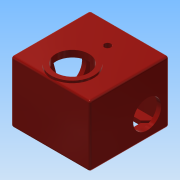
# Autodesk Inventor part: кожух  блока
Saved by Autodesk Inventor 2017 (Build 210142000, 142)
## iProperties
Part Number: кожух  блока
Material: Типовые
Document SubType Name: Modeling
Designer: Max
Mass: 1.18603 g
Surface Area: 24.9841 cm^2
Volume: 1.18603 cm^3
Density: 1 g/cm^3
Appearance: Оранжево-красный
Author: Max
Autodesk Inventor part; units mm, degrees
ref_plane "YZ Plane" through (0, 0, 0) normal (1, 0, 0) x (0, 1, 0)
ref_plane "XZ Plane" through (0, 0, 0) normal (0, 1, 0) x (-1, 0, 0)
ref_plane "XY Plane" through (0, 0, 0) normal (0, 0, 1) x (1, 0, 0)
sketch "Эскиз1" plane through (0, 0, 0) normal (0, 0, 1) x (1, 0, 0)
  line L0 (-8, -8) -> (8, -8)
  line L1 (8, -8) -> (8, 8)
  line L2 (8, 8) -> (-8, 8)
  line L3 (-8, 8) -> (-8, -8)
  circle A0 centre (0, -4) radius 2.3157
  circle A1 centre (0, 4) radius 0.75
  line L4 (-9, -9) -> (9, -9)
  line L5 (9, -9) -> (9, 9)
  line L6 (9, 9) -> (-9, 9)
  line L7 (-9, 9) -> (-9, -9)
  point P0 (0, 0)
  dimension "d0" = 16
  dimension "d1" = 16
  dimension "d2" = 8
  dimension "d3" = 8
  dimension "d4" = 1.5
  dimension "d5" = 4
  dimension "d6" = 4
  dimension "d7" = 1
  constraints: 16 end point, 4 parallel, 2 centre point, 2 perpendicular, 1 horizontal, 3 other
  measures "d0" distance between parallel lines of L1 L3
  measures "d1" distance between parallel lines of L2 L0
  measures "d2" distance from line of L0 point (0, 0)
  measures "d3" distance from line of L3 point (0, 0)
  measures "d4" diameter of A1
  measures "d5" distance from line of L0 A0.centre
  measures "d6" distance from line of L2 A1.centre
  measures "d7" distance between parallel lines of L3 L7
extrude "Выдавливание1" add sketch "Эскиз1" along normal blind 1 contours L3 L2 L1 L0 | L7 L6 L5 L4
extrude "Выдавливание2" add sketch "Эскиз1" against normal blind 13 contours L7 L6 L5 L4
sketch "Эскиз2" plane through (0, 0, -13) normal (0, 0, -1) x (-1, 0, 0)
  line L0 (-8, -8) -> (-8, 8)
  line L1 (-8, 8) -> (8, 8)
  line L2 (8, 8) -> (8, -8)
  line L3 (8, -8) -> (-8, -8)
  line L4 (-9, -9) -> (9, -9)
  line L5 (9, -9) -> (9, 9)
  line L6 (9, 9) -> (-9, 9)
  line L7 (-9, 9) -> (-9, -9)
  line L8 (-6, 5.5) -> (-6, -5.5)
  line L9 (6, -5.5) -> (6, 5.5)
  line L10 (5.5, 6) -> (-5.5, 6)
  spline S0 degree 3 number of poles 196 construction
  circle A0 centre (0, -4) radius 2.3157
  arc A1 (-1.5842, -6) -> (1.5842, -6) centre (0, -4) ccw
  line L11 (-5.5, -6) -> (-1.5842, -6)
  line L12 (-1.1537, -6) -> (-1.1341, -6)
  line L13 (1.5842, -6) -> (5.5, -6)
  line L14 (1.1397, -6) -> (1.1535, -6)
  line L15 (-8, -8) -> (8, -8) construction
  line L16 (-8, -8) -> (8, 8) construction
  line L17 (8, 8) -> (-8, 8) construction
  line L18 (-8, 8) -> (8, -8) construction
  line L19 (7.0273, 7.0273) -> (-7.0273, 7.0273) construction
  line L20 (-7.0273, 7.0273) -> (-7.0273, -7.0273) construction
  line L21 (-7.0273, -7.0273) -> (7.0273, -7.0273) construction
  line L22 (7.0273, -7.0273) -> (7.0273, 7.0273) construction
  line L23 (7.0273, 7.0273) -> (-7.0273, -7.0273) construction
  line L24 (-7.0273, 7.0273) -> (7.0273, -7.0273) construction
  arc A2 (-7.0273, -6.5273) -> (-6.5273, -7.0273) centre (-7.0273, -7.0273) ccw
  arc A3 (-6.5273, 7.0273) -> (-7.0273, 6.5273) centre (-7.0273, 7.0273) ccw
  arc A4 (7.0273, 6.5273) -> (6.5273, 7.0273) centre (7.0273, 7.0273) ccw
  arc A5 (6.5273, -7.0273) -> (7.0273, -6.5273) centre (7.0273, -7.0273) ccw
  line L25 (-6, -5.5) -> (-7.0273, -6.5273)
  line L26 (-6.5273, -7.0273) -> (-5.5, -6)
  line L27 (-6, 5.5) -> (-7.0273, 6.5273)
  line L28 (-6.5273, 7.0273) -> (-5.5, 6)
  line L29 (6.5273, -7.0273) -> (5.5, -6)
  line L30 (0, -0.5) -> (-0.5, 0)
  line L31 (0, 0.5) -> (0.5, 0)
  line L32 (6, -5.5) -> (7.0273, -6.5273)
  line L33 (0, -0.5) -> (0.5, 0)
  line L34 (6, 5.5) -> (7.0273, 6.5273)
  line L35 (6.5273, 7.0273) -> (5.5, 6)
  line L36 (0, 0.5) -> (-0.5, 0)
  point P0 (0, 0)
  dimension "d12" = 2
  dimension "d16" = 1
  dimension "d17" = 1
  dimension "d18" = 1
  dimension "d19" = 1
  constraints: 54 end point, 10 point on circle, 9 point on line, 5 centre point, 5 coincident, 2 midpoint, 2 parallel, 2 perpendicular, 1 horizontal, 4 other
  measures "d12" distance between parallel lines of L0 L8
  measures "d16" diameter of A2
  measures "d17" diameter of A3
  measures "d18" diameter of A4
  measures "d19" diameter of A5
extrude "Выдавливание3" add sketch "Эскиз2" against normal blind 1 contours L0 L1 L2 L3
fillet "Сопряжение1" radius 0.5 12 edges at (9, -9, -6) (-9, -9, -6) (-9, 9, -6) (9, 9, -6) (-9, 0, 1) (0, -9, 1) (0, 9, 1) (9, 0, 1) (0, 9, -13) (9, 0, -13) (0, -9, -13) (-9, 0, -13)
sketch "Эскиз3" plane through (0, 0, 1) normal (0, 0, 1) x (1, 0, 0)
  circle A0 centre (0, -4) radius 2.3157 projected
  circle A1 centre (0, -4) radius 2.3157
  circle A2 centre (0, -4) radius 3.75
  circle A3 centre (0, -4) radius 4.8299
  point P0 (0, 0)
  dimension "d22" = 7.5
  constraints: 3 centre point, 2 coincident
  measures "d22" diameter of A2
extrude "Выдавливание4" add sketch "Эскиз3" along normal mid plane 1 contours A3
extrude "Выдавливание5" cut sketch "Эскиз3" against normal blind 1 contours A2
sketch "Эскиз4" plane through (-9, -8.5, 0.5) normal (-1, 0, 0) x (0, 0, 1)
  circle A0 centre (-8.5, 12.5) radius 3.2 projected
  circle A1 centre (-3, 9.5) radius 1.7 projected
  line L0 (-3.8644, 8.0362) -> (-3.6612, 7.9162)
  line L1 (-3.6612, 7.9162) -> (-9.3151, 9.4056)
  line L2 (-1.8523, 10.7541) -> (-6.3396, 14.8607)
  point P0 (-0.5, 8.5)
  constraints: 6 end point, 5 tangent, 4 point on circle
extrude "Выдавливание6" cut sketch "Эскиз4" against normal blind 20 contours A0
extrude "Выдавливание7" cut sketch "Эскиз4" against normal blind 2
